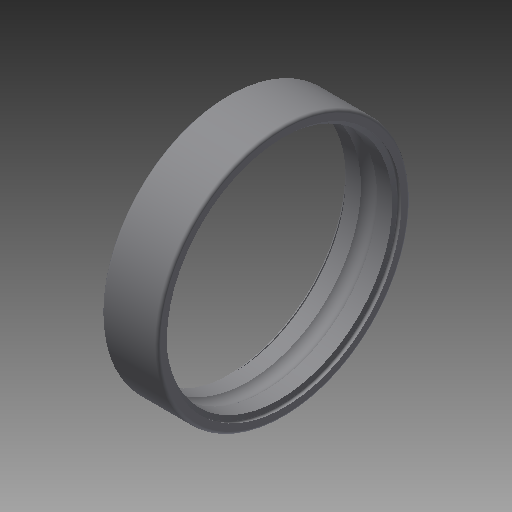
# Autodesk Inventor part: W 61701_PART2
Saved by Autodesk Inventor 2018.3 (Build 223284000, 284)
## iProperties
Category: PARTsolutions
Company: SKF
Created: 2018-07-20
Part Number: W 61701_PART2
Material: Generic
Catalog Web Link: www.cadenas.de
Description: -Deep groove ball bearings, stainless steel, single row
Vendor: SKF
Document SubType Name: Modeling
Designer: psadmin
Manufacturer: SKF
Mass: 0.180226 g
Surface Area: 5.39602 cm^2
Volume: 0.180226 cm^3
Density: 1 g/cm^3
Appearance: PSOLRGB-175-175-175
PSOL_IDENT_0: {$CADENAS_DATA\23d-libs\skf\bearings_units_and_housings\ball_bearings\deep_groove_ball_bearings\deep
PSOL_IDENT_1: _groove_ball_bearings_stainless_steel\bb1_004_104.prj},193 {VTYP=3D},{NB=W 61701_PART2},{LINA=W 6170
PSOL_IDENT_2: 1_PART2},{NN=BB1_004_104_PART2},{NOPRJ=TRUE},{DATE=13.07.2018 14:28:03},{GEOMDATE=26.07.2017 12:34:5
PSOL_IDENT_3: 6},{VERSION=},{LINEID=79900},{WBVAR=},{WBNUMERIC=}  {NB=W 61701_PART2},{LINA=W 61701_PART2},{KT=DUMM
PSOL_IDENT_4: Y},{PRODUCTID=},{DESIGNATION=W 61701},{DD=12.000},{D=18.000},{B=4.000},{DD1=13.860},{DD2=MIN},{D1=16
PSOL_IDENT_5: .100},{D2=16.700},{R12A=0.200},{LOAD1=0.527},{LOAD2=0.265},{LOAD3=0.011},{SPEED1=48000},{SPEED2=},{M
PSOL_IDENT_6: ASS=0.003},{PITCH=15.000},{DW=1.588},{Z=13.000},{II=1.000},{TYPEID=MIN},{YALG=6.93},{HALG=0.93},{HEL
PSOL_IDENT_7: P=0.95},{HELP2=0.65},{YALG1=8.05},{HALG1=0.95},{TAXONOMY=2},{DESIGN=dgbbw},{MAPPING=BCZ50,DESIGNATIO
PSOL_IDENT_8: N|IRD01,DD|ORD10,D|BCW30,B|IRD30,DD1|ORD30,D1|ORD43,D2|IRD43,DD2|ORR20,R12A|BCC02,LOAD1|BCC16,LOAD2|
PSOL_IDENT_9: BCC12,LOAD3|BCC45,SPEED1|BCM01,MASS|BCD50,PITCH|RBD10,DW|BCN81,Z|BCN80,II},{DESIGNLIST=dgbbw2z,dgbbw
PSOL_IDENT_10: ,dgbbw2rs},{SH=6.93},{SORT=DD},{RHELP=0.2},{PIM=W 61701},{R12=0.2},{HIDE=MIN}
NT: Deep groove ball bearings, stainless steel, single row
NB: W 61701_PART2
NBSYN: $DESIGNATION._PART2
LINA: W 61701_PART2
SUPPLIER: SKF
ARTICLENO: W 61701_PART2
BOMINFO: W 61701_PART2
CREATOR: CADENAS GmbH
Title: W 61701_PART2
Author: Cadenas PARTsolutions
Comments: Deep groove ball bearings, stainless steel, single row
Autodesk Inventor part; units mm, degrees
ref_plane "YZ Plane" through (0, 0, 0) normal (1, 0, 0) x (0, 1, 0)
ref_plane "XZ Plane" through (0, 0, 0) normal (0, 1, 0) x (-1, 0, 0)
ref_plane "XY Plane" through (0, 0, 0) normal (0, 0, 1) x (1, 0, 0)
sketch "Sketch_2" plane through (0, 0, 0) normal (0, 0, 1) x (1, 0, 0)
  line L0 (50, 0) -> (-50, 0)
  line L1 (0, 8.35) -> (0.06, 8.35)
  arc A0 (0.3, 8.35) -> (0.06, 8.35) centre (0.18, 8.35) ccw
  line L2 (0.3, 8.35) -> (0.3529, 8.05)
  line L3 (0.3529, 8.05) -> (1.4273, 8.05)
  arc A1 (2.5727, 8.05) -> (1.4273, 8.05) centre (2, 7.5) ccw
  line L4 (2.5727, 8.05) -> (3.6471, 8.05)
  line L5 (3.6471, 8.05) -> (3.7, 8.35)
  arc A2 (3.94, 8.35) -> (3.7, 8.35) centre (3.82, 8.35) ccw
  line L6 (3.94, 8.35) -> (4, 8.35)
  line L7 (4, 8.35) -> (4, 8.8)
  arc A3 (4, 8.8) -> (3.8, 9) centre (3.8, 8.8) ccw
  line L8 (3.8, 9) -> (0.2, 9)
  arc A4 (0.2, 9) -> (0, 8.8) centre (0.2, 8.8) ccw
  line L9 (0, 8.8) -> (0, 8.35)
  constraints: 20 end point, 10 point on circle, 5 centre point
revolve "Revolution1" add sketch "Sketch_2" angle 360 about axis through (50, 0, 0) along (1, 0, 0)
body "Solid1"
